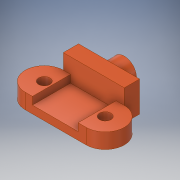
# Autodesk Inventor part: КВ33.044.206 - Крепеж держателя ремня
Saved by Autodesk Inventor 2019 (Build 230136000, 136)
## iProperties
Created: 2019-08-18
Part Number: КВ33.044.206 - Крепеж держателя ремня
Material: Пластик АБС
Document SubType Name: Modeling
Designer: Петров Иван
Density: 1.06 g/cm^3
Appearance: Гладкий — светло-оранжевый
Author: Петров Иван
Autodesk Inventor part; units mm, degrees
ref_plane "YZ Plane" through (0, 0, 0) normal (1, 0, 0) x (0, 1, 0)
ref_plane "XZ Plane" through (0, 0, 0) normal (0, 1, 0) x (-1, 0, 0)
ref_plane "XY Plane" through (0, 0, 0) normal (0, 0, 1) x (1, 0, 0)
sketch "Эскиз1" plane through (0, 0, 0) normal (0, 0, 1) x (1, 0, 0)
  line L0 (-4, -1) -> (4, -1)
  line L1 (4, -1) -> (4, 1)
  line L2 (4, 1) -> (-4, 1)
  line L3 (-4, 1) -> (-4, -1)
  line L4 (-4, -1) -> (4, 1) construction
  line L5 (4, -1) -> (-4, 1) construction
  point P0 (0, 0)
  dimension "d0" = 8
  dimension "d1" = 2
  constraints: 12 end point, 2 midpoint, 2 parallel, 1 horizontal, 1 perpendicular
  measures "d0" distance of L2.end L1.end
  measures "d1" distance of L1.end L0.end
extrude "Выдавливание1" add sketch "Эскиз1" along normal blind 5
sketch "Эскиз2" plane through (-4, 1, 0) normal (0, 1, 0) x (1, 0, 0)
  line L0 (0, 0) -> (0, -5) projected
  circle A0 centre (0, -2.5) radius 2.5
  line L1 (8, 0) -> (8, -5) projected
  circle A1 centre (8, -2.5) radius 2.5
  point P0 (4, 0)
  dimension "d4" = 5
  dimension "d5" = 5
  constraints: 2 centre point, 2 midpoint
  measures "d4" diameter of A0
  measures "d5" diameter of A1
extrude "Выдавливание2" add sketch "Эскиз2" against normal blind 2
sketch "Эскиз3" plane through (-4, 1, 0) normal (0, 1, 0) x (1, 0, 0)
  arc A0 (0, 0) -> (0, -5) centre (0, -2.5) ccw projected
  circle A1 centre (0, -2.5) radius 0.75
  arc A2 (8, -5) -> (8, 0) centre (8, -2.5) ccw projected
  circle A3 centre (8, -2.5) radius 0.75
  point P0 (4, 0)
  dimension "d8" = 1.5
  dimension "d9" = 1.5
  constraints: 2 centre point, 2 coincident
  measures "d8" diameter of A1
  measures "d9" diameter of A3
extrude "Выдавливание3" cut sketch "Эскиз3" against normal blind 2
sketch "Эскиз4" plane through (-4, 1, 0) normal (0, 1, 0) x (1, 0, 0)
  line L0 (4, 0) -> (4, -5)
  line L1 (0, -5) -> (8, -5) projected
  line L2 (0, 0) -> (8, 0) projected
  line L3 (6.9421, -5) -> (0.9421, -5)
  line L4 (0.9421, -5) -> (0.9421, 0)
  line L5 (0.9421, 0) -> (6.9421, 0)
  line L6 (6.9421, 0) -> (6.9421, -5)
  line L7 (6.9421, -5) -> (0.9421, 0) construction
  line L8 (0.9421, -5) -> (6.9421, 0) construction
  point P0 (3.9421, -2.5)
  dimension "d12" = 6
  constraints: 14 end point, 3 midpoint, 2 parallel, 1 horizontal, 1 perpendicular, 1 point on line
  measures "d12" distance of L4.end L5.end
extrude "Выдавливание4" cut sketch "Эскиз4" against normal blind 1
sketch "Эскиз5" plane through (0, 0, 0) normal (0, 0, -1) x (-1, 0, 0)
  line L0 (-3.25, -1) -> (-4.75, -1) projected
  line L1 (-4, -1) -> (4, -1)
  line L2 (4, -1) -> (4, 3)
  line L3 (4, 3) -> (-4, 3)
  line L4 (-4, 3) -> (-4, -1)
  point P0 (0, 0)
  dimension "d15" = 8
  dimension "d16" = 4
  constraints: 8 end point, 2 parallel, 1 horizontal, 1 midpoint, 1 perpendicular
  measures "d15" distance of L3.end L2.end
  measures "d16" distance of L1.end L2.end
extrude "Выдавливание5" add sketch "Эскиз5" along normal blind 2
sketch "Эскиз6" plane through (0, 0, -2) normal (0, 0, -1) x (-1, 0, 0)
  line L0 (-4, 3) -> (-4, 1) projected
  line L1 (-4, 1) -> (4, 1)
  line L2 (3.25, 1) -> (4.75, 1) projected
  circle A0 centre (0, 1) radius 1.25
  circle A1 centre (0, 1) radius 1.6
  point P0 (0, 0)
  dimension "d19" = 2.5
  dimension "d20" = 3.2
  constraints: 2 centre point, 2 end point, 2 midpoint, 1 coincident
  measures "d19" diameter of A0
  measures "d20" diameter of A1
extrude "Выдавливание6" add sketch "Эскиз6" along normal blind 2 contours A0 L1 A1 | L1 A1 A0
sketch "Эскиз7" plane through (-4, 1, 5) normal (0, 1, 0) x (1, 0, 0)
  circle A0 centre (0, 2.5) radius 0.75 projected
  line L0 (0.9421, 0) -> (0.9421, 5) projected
  line L1 (0.9421, 5) -> (0, 5) projected
  arc A1 (0, 5) -> (0, 0) centre (0, 2.5) ccw projected
  line L2 (0.9421, 0) -> (0, 0) projected
  line L3 (0.9421, 0) -> (0.9421, 5) projected
  line L4 (6.9421, 0) -> (0.9421, 0) projected
  line L5 (6.9421, 5) -> (6.9421, 0) projected
  line L6 (0.9421, 5) -> (6.9421, 5) projected
  circle A2 centre (8, 2.5) radius 0.75 projected
  line L7 (6.9421, 5) -> (6.9421, 0) projected
  line L8 (8, 0) -> (6.9421, 0) projected
  arc A3 (8, 0) -> (8, 5) centre (8, 2.5) ccw projected
  line L9 (8, 5) -> (6.9421, 5) projected
  point P0 (4, 5)
